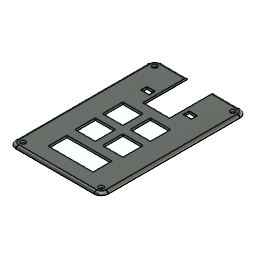
top (Autodesk Fusion 360 design; units mm, degrees)
part number: 2025-12-17-17-08-39-744
Autodesk Fusion 360 part; units mm, degrees
sketch "plate-2025-12-17T11_17_56.332Z" plane through (0, 0, 0) normal (0, 0, 1) x (1, 0, 0)
  line L0 (3.025, -11.575) -> (16.025, -11.575)
  line L1 (3.025, -25.575) -> (16.025, -25.575)
  line L2 (2.525, -12.075) -> (2.525, -25.075)
  line L3 (16.525, -12.075) -> (16.525, -25.075)
  arc A0 (3.025, -11.575) -> (2.525, -12.075) centre (3.025, -12.075) ccw
  arc A1 (16.525, -12.075) -> (16.025, -11.575) centre (16.025, -12.075) ccw
  arc A2 (2.525, -25.075) -> (3.025, -25.575) centre (3.025, -25.075) ccw
  arc A3 (16.025, -25.575) -> (16.525, -25.075) centre (16.025, -25.075) ccw
  line L4 (22.075, -11.575) -> (35.075, -11.575)
  line L5 (22.075, -25.575) -> (35.075, -25.575)
  line L6 (21.575, -12.075) -> (21.575, -25.075)
  line L7 (35.575, -12.075) -> (35.575, -25.075)
  arc A4 (22.075, -11.575) -> (21.575, -12.075) centre (22.075, -12.075) ccw
  arc A5 (35.575, -12.075) -> (35.075, -11.575) centre (35.075, -12.075) ccw
  arc A6 (21.575, -25.075) -> (22.075, -25.575) centre (22.075, -25.075) ccw
  arc A7 (35.075, -25.575) -> (35.575, -25.075) centre (35.075, -25.075) ccw
  line L8 (3.025, -30.625) -> (16.025, -30.625)
  line L9 (3.025, -44.625) -> (16.025, -44.625)
  line L10 (2.525, -31.125) -> (2.525, -44.125)
  line L11 (16.525, -31.125) -> (16.525, -44.125)
  arc A8 (3.025, -30.625) -> (2.525, -31.125) centre (3.025, -31.125) ccw
  arc A9 (16.525, -31.125) -> (16.025, -30.625) centre (16.025, -31.125) ccw
  arc A10 (2.525, -44.125) -> (3.025, -44.625) centre (3.025, -44.125) ccw
  arc A11 (16.025, -44.625) -> (16.525, -44.125) centre (16.025, -44.125) ccw
  line L12 (22.075, -30.625) -> (35.075, -30.625)
  line L13 (22.075, -44.625) -> (35.075, -44.625)
  line L14 (21.575, -31.125) -> (21.575, -44.125)
  line L15 (35.575, -31.125) -> (35.575, -44.125)
  arc A12 (22.075, -30.625) -> (21.575, -31.125) centre (22.075, -31.125) ccw
  arc A13 (35.575, -31.125) -> (35.075, -30.625) centre (35.075, -31.125) ccw
  arc A14 (21.575, -44.125) -> (22.075, -44.625) centre (22.075, -44.125) ccw
  arc A15 (35.075, -44.625) -> (35.575, -44.125) centre (35.075, -44.125) ccw
sketch "Sketch2" plane through (0, 0, 0) normal (0, 0, 1) x (1, 0, 0)
  line L0 (-12.875, 25.875) -> (51.125, 25.875)
  line L1 (51.125, 25.875) -> (51.125, -75.125)
  line L2 (51.125, -75.125) -> (-12.875, -75.125)
  line L3 (-12.875, -75.125) -> (-12.875, 25.875)
  line L4 (3.025, -44.625) -> (16.025, -44.625)
  line L5 (2.525, -12.075) -> (2.525, -25.075)
  line L6 (9.875, 25.875) -> (28.375, 25.875)
  line L7 (28.375, 25.875) -> (28.375, -5.125)
  line L8 (28.375, -5.125) -> (9.875, -5.125)
  line L9 (9.875, -5.125) -> (9.875, 25.875)
  line L10 (3.125, -50.7993) -> (34.125, -50.7993)
  line L11 (34.125, -50.7993) -> (34.125, -63.7993)
  line L12 (34.125, -63.7993) -> (3.125, -63.7993)
  line L13 (3.125, -63.7993) -> (3.125, -50.7993)
  circle A0 centre (46.125, 20.875) radius 1.7
  circle A1 centre (46.125, -70.125) radius 1.7
  circle A2 centre (-7.875, -70.125) radius 1.7
  circle A3 centre (-7.875, 20.875) radius 1.7
  dimension "d1" = 101
  dimension "d2" = 64
  dimension "d3" = 30.5
  dimension "d4" = 15.4
  dimension "d5" = 31
  dimension "d6" = 18.5
  dimension "d7" = 22.75
  dimension "d8" = 13
  dimension "d9" = 31
  dimension "d10" = 16
  dimension "d11" = 3.4
  dimension "d12" = 5
  dimension "d13" = 5
  dimension "d14" = 3.4
  dimension "d15" = 3.4
  dimension "d16" = 3.4
  constraint horizontal L0
  constraint vertical L1
  constraint horizontal L2
  constraint vertical L3
  constraint horizontal L6
  constraint vertical L7
  constraint horizontal L8
  constraint vertical L9
  constraint coincident L0 L6.start
  constraint horizontal L10
  constraint vertical L11
  constraint horizontal L12
  constraint vertical L13
  measures "d1" distance of L0 L2
  measures "d2" distance of L1 L3
  measures "d3" distance of L2 L4
  measures "d4" distance of L3 L5
  measures "d5" distance of L6.start L8.end
  measures "d6" distance of L7 L9
  measures "d7" distance of L3 L9
  measures "d8" distance of L10.start L12.end
  measures "d9" distance of L11 L13
  measures "d10" distance of L3 L13
  measures "d11" diameter of A0
  measures "d12" distance of L1 A0.centre
  measures "d13" distance of L0 A0.centre
  measures "d14" diameter of A1
  measures "d15" diameter of A2
  measures "d16" diameter of A3
extrude "Extrude1" add sketch "Sketch2" along normal blind 1.5 contours L0 L1 L2 L3 L7 L8 L9
extrude "Extrude2" cut sketch "plate-2025-12-17T11_17_56.332Z" along normal blind 1.5
fillet "Fillet1" radius 5 1 edges at (51.125, -75.125, 0.75)
fillet "Fillet2" radius 5 1 edges at (51.125, 25.875, 0.75)
fillet "Fillet3" radius 5 1 edges at (-12.875, -75.125, 0.75)
fillet "Fillet4" radius 5 1 edges at (-12.875, 25.875, 0.75)
fillet "Fillet5" radius 2 9 edges at (1, 25.875, 1.5) (-11.4105, 24.4105, 1.5) (-12.875, -24.625, 1.5) (-11.4105, -73.6605, 1.5) (19.125, -75.125, 1.5) (49.6605, -73.6605, 1.5) (51.125, -24.625, 1.5) (49.6605, 24.4105, 1.5) (37.25, 25.875, 1.5)
sketch "Sketch3" plane through (0, 0, 1.5) normal (0, 0, 1) x (-1, 0, 0)
  line L0 (-34.125, 63.7993) -> (-3.125, 63.7993)
  line L1 (-3.125, 63.7993) -> (-3.125, 50.7993)
  line L2 (-3.125, 50.7993) -> (-34.125, 50.7993)
  line L3 (-34.125, 50.7993) -> (-34.125, 63.7993)
  circle A0 centre (7.875, 70.125) radius 1.7
  circle A1 centre (-46.125, -20.875) radius 1.7
  circle A2 centre (7.875, -20.875) radius 1.7
  circle A3 centre (-46.125, 70.125) radius 1.7
  line L4 (-3.025, 11.575) -> (-16.025, 11.575)
  arc A4 (-16.525, 12.075) -> (-16.025, 11.575) centre (-16.025, 12.075) ccw
  line L5 (-16.525, 12.075) -> (-16.525, 25.075)
  arc A5 (-16.025, 25.575) -> (-16.525, 25.075) centre (-16.025, 25.075) ccw
  line L6 (-16.025, 25.575) -> (-3.025, 25.575)
  arc A6 (-2.525, 25.075) -> (-3.025, 25.575) centre (-3.025, 25.075) ccw
  line L7 (-2.525, 25.075) -> (-2.525, 12.075)
  arc A7 (-3.025, 11.575) -> (-2.525, 12.075) centre (-3.025, 12.075) ccw
  line L8 (-3.025, 30.625) -> (-16.025, 30.625)
  arc A8 (-16.525, 31.125) -> (-16.025, 30.625) centre (-16.025, 31.125) ccw
  line L9 (-16.525, 31.125) -> (-16.525, 44.125)
  arc A9 (-16.025, 44.625) -> (-16.525, 44.125) centre (-16.025, 44.125) ccw
  line L10 (-16.025, 44.625) -> (-3.025, 44.625)
  arc A10 (-2.525, 44.125) -> (-3.025, 44.625) centre (-3.025, 44.125) ccw
  line L11 (-2.525, 44.125) -> (-2.525, 31.125)
  arc A11 (-3.025, 30.625) -> (-2.525, 31.125) centre (-3.025, 31.125) ccw
  line L12 (-22.075, 11.575) -> (-35.075, 11.575)
  arc A12 (-35.575, 12.075) -> (-35.075, 11.575) centre (-35.075, 12.075) ccw
  line L13 (-35.575, 12.075) -> (-35.575, 25.075)
  arc A13 (-35.075, 25.575) -> (-35.575, 25.075) centre (-35.075, 25.075) ccw
  line L14 (-35.075, 25.575) -> (-22.075, 25.575)
  arc A14 (-21.575, 25.075) -> (-22.075, 25.575) centre (-22.075, 25.075) ccw
  line L15 (-21.575, 25.075) -> (-21.575, 12.075)
  arc A15 (-22.075, 11.575) -> (-21.575, 12.075) centre (-22.075, 12.075) ccw
  line L16 (-22.075, 30.625) -> (-35.075, 30.625)
  arc A16 (-35.575, 31.125) -> (-35.075, 30.625) centre (-35.075, 31.125) ccw
  line L17 (-35.575, 31.125) -> (-35.575, 44.125)
  arc A17 (-35.075, 44.625) -> (-35.575, 44.125) centre (-35.075, 44.125) ccw
  line L18 (-35.075, 44.625) -> (-22.075, 44.625)
  arc A18 (-21.575, 44.125) -> (-22.075, 44.625) centre (-22.075, 44.125) ccw
  line L19 (-21.575, 44.125) -> (-21.575, 31.125)
  arc A19 (-22.075, 30.625) -> (-21.575, 31.125) centre (-22.075, 31.125) ccw
  line L20 (-9.875, -23.9385) -> (7.875, -23.9385)
  arc A20 (7.875, -23.9385) -> (10.9385, -20.875) centre (7.875, -20.875) ccw
  line L21 (10.9385, -20.875) -> (10.9385, 70.125)
  arc A21 (10.9385, 70.125) -> (7.875, 73.1885) centre (7.875, 70.125) ccw
  line L22 (7.875, 73.1885) -> (-46.125, 73.1885)
  arc A22 (-46.125, 73.1885) -> (-49.1885, 70.125) centre (-46.125, 70.125) ccw
  line L23 (-49.1885, 70.125) -> (-49.1885, -20.875)
  arc A23 (-49.1885, -20.875) -> (-46.125, -23.9385) centre (-46.125, -20.875) ccw
  line L24 (-46.125, -23.9385) -> (-28.375, -23.9385)
  line L25 (-28.375, -23.9385) -> (-28.375, 5.125)
  line L26 (-28.375, 5.125) -> (-9.875, 5.125)
  line L27 (-9.875, 5.125) -> (-9.875, -23.9385)
sketch "Sketch4" plane through (0, 0, 0) normal (0, 0, 1) x (1, 0, 0)
  line L0 (36.475, 1.875) -> (30.875, 1.875)
  line L1 (30.875, 1.875) -> (30.875, 5.875)
  line L2 (30.875, 5.875) -> (36.475, 5.875)
  line L3 (36.475, 5.875) -> (36.475, 1.875)
  line L4 (28.375, 25.875) -> (46.125, 25.875)
  line L5 (7.275, 5.875) -> (7.275, 1.875)
  line L6 (7.275, 1.875) -> (1.675, 1.875)
  line L7 (1.675, 5.875) -> (7.275, 5.875)
  line L8 (1.675, 1.875) -> (1.675, 5.875)
  line L9 (28.375, 23.9385) -> (28.375, -5.125)
  line L10 (9.875, -5.125) -> (9.875, 23.9385)
  dimension "d31" = 5.6
  dimension "d32" = 20
  dimension "d33" = 5.6
  dimension "d34" = 2.5
  dimension "d35" = 2.6
  constraint horizontal L0
  constraint vertical L1
  constraint horizontal L2
  constraint vertical L3
  constraint horizontal L6
  constraint vertical L8
  constraint horizontal L7
  constraint vertical L5
  measures "d31" distance of L1 L3
  measures "d32" distance of L2 L4
  measures "d33" distance of L5 L8
  measures "d34" distance of L1 L9
  measures "d35" distance of L5 L10
extrude "Extrude3" cut sketch "Sketch4" along normal blind 1.5
sketch "Sketch5" plane through (0, 0, 0) normal (0, 0, 1) x (1, 0, 0)
sketch "Sketch6" plane through (0, 0, 0) normal (0, 0, 1) x (1, 0, 0)
